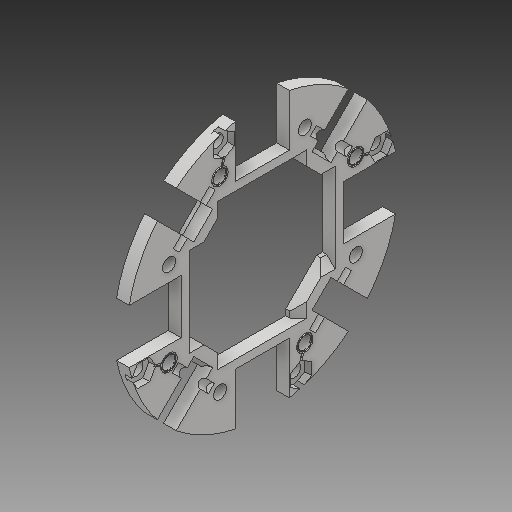
# Autodesk Inventor part: deska
Saved by Autodesk Inventor 2018 (Build 220112000, 112)
## iProperties
Created: 2018-03-10
Part Number: deska
Material: Všeobecné
Document SubType Name: Modeling
Designer: Kuba
Density: 1 g/cm^3
Appearance: Výchozí
Mass: 3.41348 g
Surface Area: 43.4622 cm^2
Volume: 3.41348 cm^3
Author: Kuba
Autodesk Inventor part; units mm, degrees
ref_plane "YZ Plane" through (0, 0, 0) normal (1, 0, 0) x (0, 1, 0)
sketch "Náčrt1" plane through (0, 0, 0) normal (1, 0, 0) x (0, 1, 0)
  line L0 (19.1636, 6.35) -> (31.3636, 6.35)
  line L1 (31.3636, -6.35) -> (19.1636, -6.35)
  line L2 (19.1636, -6.35) -> (19.1636, 6.35)
  line L3 (24.7449, 20.2901) -> (16.7231, 12.2683)
  line L4 (16.7231, 12.2683) -> (12.2683, 16.7231)
  line L5 (12.2683, 16.7231) -> (20.2901, 24.7449)
  line L6 (0, 0) -> (14.4957, 14.4957)
  line L7 (6.35, 19.1636) -> (-6.35, 19.1636)
  line L8 (6.35, 31.3636) -> (6.35, 19.1636)
  line L9 (-6.35, 19.1636) -> (-6.35, 31.3636)
  line L10 (-20.2901, 24.7449) -> (-12.2683, 16.7231)
  line L11 (-12.2683, 16.7231) -> (-16.7231, 12.2683)
  line L12 (-16.7231, 12.2683) -> (-24.7449, 20.2901)
  line L13 (-19.1636, 6.35) -> (-19.1636, -6.35)
  line L14 (-31.3636, 6.35) -> (-19.1636, 6.35)
  line L15 (-19.1636, -6.35) -> (-31.3636, -6.35)
  line L16 (-24.7449, -20.2901) -> (-16.7231, -12.2683)
  line L17 (-16.7231, -12.2683) -> (-12.2683, -16.7231)
  line L18 (-12.2683, -16.7231) -> (-20.2901, -24.7449)
  line L19 (-6.35, -19.1636) -> (6.35, -19.1636)
  line L20 (-6.35, -31.3636) -> (-6.35, -19.1636)
  line L21 (6.35, -19.1636) -> (6.35, -31.3636)
  line L22 (20.2901, -24.7449) -> (12.2683, -16.7231)
  line L23 (12.2683, -16.7231) -> (16.7231, -12.2683)
  line L24 (16.7231, -12.2683) -> (24.7449, -20.2901)
  arc A0 (24.7449, -20.2901) -> (31.3636, -6.35) centre (0, 0) ccw
  arc A1 (6.35, -31.3636) -> (20.2901, -24.7449) centre (0, 0) ccw
  arc A2 (-20.2901, -24.7449) -> (-6.35, -31.3636) centre (0, 0) ccw
  arc A3 (-31.3636, -6.35) -> (-24.7449, -20.2901) centre (0, 0) ccw
  arc A4 (-24.7449, 20.2901) -> (-31.3636, 6.35) centre (0, 0) ccw
  arc A5 (-6.35, 31.3636) -> (-20.2901, 24.7449) centre (0, 0) ccw
  arc A6 (31.3636, 6.35) -> (24.7449, 20.2901) centre (0, 0) ccw
  arc A7 (20.2901, 24.7449) -> (6.35, 31.3636) centre (0, 0) ccw
  line L25 (16.2792, 20.734) -> (20.734, 16.2792)
  line L26 (14.9711, 23.4564) -> (13.5569, 22.0421)
  line L27 (13.5569, 22.0421) -> (22.0421, 13.5569)
  line L28 (22.0421, 13.5569) -> (23.4564, 14.9711)
  line L29 (23.4564, 14.9711) -> (14.9711, 23.4564)
  line L30 (-13.5569, 22.0421) -> (-14.9711, 23.4564)
  line L31 (-22.0421, 13.5569) -> (-13.5569, 22.0421)
  line L32 (-14.9711, 23.4564) -> (-23.4564, 14.9711)
  line L33 (-23.4564, 14.9711) -> (-22.0421, 13.5569)
  line L34 (-22.0421, -13.5569) -> (-23.4564, -14.9711)
  line L35 (-13.5569, -22.0421) -> (-22.0421, -13.5569)
  line L36 (-23.4564, -14.9711) -> (-14.9711, -23.4564)
  line L37 (-14.9711, -23.4564) -> (-13.5569, -22.0421)
  line L38 (13.5569, -22.0421) -> (14.9711, -23.4564)
  line L39 (22.0421, -13.5569) -> (13.5569, -22.0421)
  line L40 (14.9711, -23.4564) -> (23.4564, -14.9711)
  line L41 (23.4564, -14.9711) -> (22.0421, -13.5569)
  line L42 (0, 0) -> (2.9116, 0)
  point P0 (-14.4957, 14.4957)
  point P1 (-14.4957, -14.4957)
  point P2 (14.4957, -14.4957)
  dimension "d1" = 6.35
  dimension "d2" = 6.35
  dimension "d4" = 6.3
  dimension "d5" = 3.15
  dimension "d6" = 20.5
  dimension "d7" = 45
  dimension "d10" = 360
  dimension "d12" = 2
  dimension "d13" = 12
  dimension "d14" = 1
  dimension "d15" = 2.85
  dimension "d18" = 360
  dimension "d105" = 32
  dimension "d106" = 45
  dimension "d107" = 12.2
  constraints: 86 end point, 16 point on circle, 8 centre point, 6 midpoint, 4 parallel, 3 perpendicular, 2 horizontal, 1 coincident, 94 other
  measures "d1" vertical distance of point (0, 0) L0.start
  measures "d2" distance from line of point (0, 0) L1
  measures "d4" distance between parallel lines of L3 L5
  measures "d5" distance between parallel lines of L6 L5
  measures "d6" distance from line of point (0, 0) L4
  measures "d7" angle of L2 L6
  measures "d12" distance of L26.start L26.end
  measures "d13" distance of L28.end L26.start
  measures "d14" distance between parallel lines of L25 L29
  measures "d15" distance between parallel lines of L5 L26
  measures "d105" radius of A5
  measures "d106" angle of L42 L6
  measures "d107" distance of L0.end L0.start
extrude "Vysunutí1" add sketch "Náčrt1" along normal mid plane 3 contours L2 L1 A0 L24 L40 L41 L39 L23 L22 L38 A1 L21 L19 L20 A2 L18 L36 L37 L35 L17 L16 L34 A3 L15 L13 L14 A4 L12 L32 L33 L31 L11 L10 L30 A5 L9 L7 L8 A7 L5 L29 L26 L27 L4 L3 L28 A6 L0 | L29 L28 L27 L3 | L5 L27 L26 L29 | L24 L39 L41 L40 | L40 L38 L39 L22 | L32 L30 L31 L10 | L12 L31 L33 L32 | L18 L35 L37 L36 | L36 L34 L35 L16
ref_plane "Pracovní rovina1" through (1.5, 0, 0) normal (1, 0, 0) x (0, 0, -1)
ref_plane "Pracovní rovina2" through (-1.5, 0, 0) normal (-1, 0, 0) x (0, 0, 1)
sketch "Náčrt6" plane through (-1.5, 0, 0) normal (1, 0, 0) x (0, 0, -1)
  circle A0 centre (10, 22) radius 1.3
  circle A1 centre (-10, 22) radius 1.3
  circle A2 centre (-22, 10) radius 1.3
  circle A3 centre (-22, -10) radius 1.3
  circle A4 centre (-10, -22) radius 1.3
  circle A5 centre (10, -22) radius 1.3
  circle A6 centre (22, -10) radius 1.3
  circle A7 centre (22, 10) radius 1.3
  point P0 (0, 0)
  dimension "d52" = 2.6
  dimension "d53" = 2.6
  dimension "d54" = 22
  dimension "d55" = 22
  dimension "d56" = 10
  dimension "d57" = 10
  dimension "d60" = 360
  constraints: 8 centre point, 17 other
  measures "d52" diameter of A0
  measures "d53" diameter of A1
  measures "d54" vertical distance of point (0, 0) A0.centre
  measures "d55" vertical distance of point (0, 0) A1.centre
  measures "d56" horizontal distance of point (0, 0) A0.centre
  measures "d57" horizontal distance of point (0, 0) A1.centre
sketch "Sketch7" plane through (-1.5, 16.7231, 12.2683) normal (0, -0.7071, 0.7071) x (1, 0, 0)
  circle A0 centre (2.9795, 2.3446) radius 1
  line L0 (0, 11.3446) -> (3, 11.3446) projected
  point P0 (1.5, -20.5)
  dimension "d64" = 2
  dimension "d65" = 9
  constraints: 1 centre point
  measures "d64" diameter of A0
  measures "d65" distance from line of L0 A0.centre
extrude "Extrusion6" cut sketch "Sketch7" against normal blind 3 and the other way blind 9
pattern_circular "Circular Pattern1" count 4 over 360 about axis through (0, 0, 0) along (1, 0, 0) of "Extrusion6"
hole "Hole3" at (-1.5, 10, 22) at (-1.5, 22, 10) at (-1.5, -10, 22) at (-1.5, -22, 10) at (-1.5, -22, -10) at (-1.5, 22, -10) at (-1.5, 10, -22) at (-1.5, -10, -22) direction (1, 0, 0) diameter 3.1 end through all countersink diameter 4.8 countersink angle 90
sketch "Sketch9" plane through (1.5, -20.2901, 24.7449) normal (0, -0.7071, -0.7071) x (-1, 0, 0)
  circle A0 centre (0.0205, 9) radius 3.15
  arc A1 (0, 8.0002) -> (0, 9.9998) centre (0.0205, 9) ccw projected
  point P0 (1.5, 31.8446)
  dimension "d102" = 6.3
  constraints: 1 centre point, 1 concentric
  measures "d102" diameter of A0
extrude "Extrusion7" cut sketch "Sketch9" along normal blind 6.3
pattern_circular "Circular Pattern2" count 4 over 360 about axis through (0, 0, 0) along (1, 0, 0) of "Extrusion7"
sketch "Sketch10" plane through (1.5, 0, 0) normal (1, 0, 0) x (0, 0, -1)
  line L0 (7.1094, 17.1636) -> (17.1636, 7.1094)
  line L1 (17.1636, 7.1094) -> (17.1636, -7.1094)
  line L2 (17.1636, -7.1094) -> (7.1094, -17.1636)
  line L3 (7.1094, -17.1636) -> (-7.1094, -17.1636)
  line L4 (-7.1094, -17.1636) -> (-17.1636, -7.1094)
  line L5 (-17.1636, -7.1094) -> (-17.1636, 7.1094)
  line L6 (-17.1636, 7.1094) -> (-7.1094, 17.1636)
  line L7 (-7.1094, 17.1636) -> (7.1094, 17.1636)
  line L8 (6.35, 19.1636) -> (-6.35, 19.1636) projected
  point P0 (0, 0)
  point P1 (0, 0)
  dimension "d111" = 2
  constraints: 16 end point, 1 coincident, 1 vertical, 17 other
  measures "d111" distance between parallel lines of L8 L7
extrude "Extrusion8" cut sketch "Sketch10" against normal blind 6.3
sketch "Sketch11" plane through (1.5, 0, 0) normal (1, 0, 0) x (0, 0, -1)
  line L0 (8.5, -17.1636) -> (-8.5, -17.1636)
  line L1 (-8.5, -17.1636) -> (-8.5, -7.1636)
  line L2 (-8.5, -7.1636) -> (8.5, -7.1636)
  line L3 (8.5, -7.1636) -> (8.5, -17.1636)
  line L4 (7.1094, -17.1636) -> (-7.1094, -17.1636) projected
  line L5 (0, 0) -> (0, -3.635)
  line L6 (0, 0) -> (-4.1702, 0)
  line L7 (17.1636, 8.5) -> (17.1636, -8.5)
  line L8 (17.1636, -8.5) -> (7.1636, -8.5)
  line L9 (7.1636, -8.5) -> (7.1636, 8.5)
  line L10 (7.1636, 8.5) -> (17.1636, 8.5)
  line L11 (-8.5, 17.1636) -> (8.5, 17.1636)
  line L12 (8.5, 17.1636) -> (8.5, 7.1636)
  line L13 (8.5, 7.1636) -> (-8.5, 7.1636)
  line L14 (-8.5, 7.1636) -> (-8.5, 17.1636)
  line L15 (-17.1636, -8.5) -> (-17.1636, 8.5)
  line L16 (-17.1636, 8.5) -> (-7.1636, 8.5)
  line L17 (-7.1636, 8.5) -> (-7.1636, -8.5)
  line L18 (-7.1636, -8.5) -> (-17.1636, -8.5)
  point P0 (3.635, 0)
  point P1 (0, 3.635)
  point P2 (-3.635, 0)
  dimension "d114" = 10
  dimension "d115" = 17
  dimension "d118" = 360
  constraints: 36 end point, 2 horizontal, 2 parallel, 1 collinear, 1 perpendicular, 1 vertical, 38 other
  measures "d114" distance between parallel lines of L2 L0
  measures "d115" distance of L0.start L0.end
extrude "Extrusion9" cut sketch "Sketch11" against normal through all contours L0 L1 L18 L17 L2 L9 L8 L3 | L8 L9 L2 L3 | L3 L2 L9 L13 L12 L10 L7 L8 | L18 L15 L16 L14 L13 L17 L2 L1 | L1 L2 L17 L18 | L13 L17 L16 L14 L11 L12 L10 L9 | L9 L10 L12 L13 | L13 L14 L16 L17
sketch "Sketch12" plane through (1.5, -17.1636, 8.5) normal (0, 1, 0) x (1, 0, 0)
  line L0 (0, 0) -> (0, -2)
  line L1 (0, -2) -> (-2, 0)
  line L2 (0, 0) -> (-3, 0) projected
  line L3 (-2, 0) -> (-3, 0)
  line L4 (-1.5, 8.5) -> (-3, 8.5)
  line L5 (-3, 0) -> (-3, 17) projected
  dimension "d123" = 2
  dimension "d129" = 45
  constraints: 8 end point, 3 point on line, 2 horizontal, 1 vertical
  measures "d123" distance of L0.start L0.end
  measures "d129" angle of L0 L1
extrude "Extrusion10" cut sketch "Sketch12" along normal up to surface (34.3273 mm away)
pattern_circular "Circular Pattern3" count 4 over 360 about axis through (0, 0, 0) along (1, 0, 0) of "Extrusion10"
sketch "Sketch14" plane through (1.5, 0, 0) normal (1, 0, 0) x (0, 0, -1)
  line L0 (25.1132, 9.1) -> (26.5566, 11.6)
  line L1 (26.5566, 11.6) -> (29.4434, 11.6)
  line L2 (29.4434, 11.6) -> (30.8868, 9.1)
  line L3 (30.8868, 9.1) -> (29.4434, 6.6)
  line L4 (29.4434, 6.6) -> (26.5566, 6.6)
  line L5 (26.5566, 6.6) -> (25.1132, 9.1)
  line L6 (19.1636, 6.35) -> (31.3636, 6.35) projected
  line L7 (-9.1, 25.1132) -> (-11.6, 26.5566)
  line L8 (-11.6, 26.5566) -> (-11.6, 29.4434)
  line L9 (-11.6, 29.4434) -> (-9.1, 30.8868)
  line L10 (-9.1, 30.8868) -> (-6.6, 29.4434)
  line L11 (-6.6, 29.4434) -> (-6.6, 26.5566)
  line L12 (-6.6, 26.5566) -> (-9.1, 25.1132)
  line L13 (-25.1132, -9.1) -> (-26.5566, -11.6)
  line L14 (-26.5566, -11.6) -> (-29.4434, -11.6)
  line L15 (-29.4434, -11.6) -> (-30.8868, -9.1)
  line L16 (-30.8868, -9.1) -> (-29.4434, -6.6)
  line L17 (-29.4434, -6.6) -> (-26.5566, -6.6)
  line L18 (-26.5566, -6.6) -> (-25.1132, -9.1)
  line L19 (9.1, -25.1132) -> (11.6, -26.5566)
  line L20 (11.6, -26.5566) -> (11.6, -29.4434)
  line L21 (11.6, -29.4434) -> (9.1, -30.8868)
  line L22 (9.1, -30.8868) -> (6.6, -29.4434)
  line L23 (6.6, -29.4434) -> (6.6, -26.5566)
  line L24 (6.6, -26.5566) -> (9.1, -25.1132)
  point P0 (0, 0)
  point P1 (28, 9.1)
  point P2 (-9.1, 28)
  point P3 (-28, -9.1)
  point P4 (9.1, -28)
  dimension "d140" = 9.1
  dimension "d141" = 28
  dimension "d142" = 5
  dimension "d145" = 360
  constraints: 48 end point, 1 parallel, 66 other
  measures "d140" vertical distance of point (28, 9.1) point (0, 0)
  measures "d141" horizontal distance of point (0, 0) point (28, 9.1)
  measures "d142" distance between parallel lines of L4 L1
extrude "Extrusion12" cut sketch "Sketch14" against normal blind 1.6
sketch "Sketch15" plane through (1.5, 0, 0) normal (1, 0, 0) x (0, 0, -1)
  circle A0 centre (22, 10) radius 1.65
  line L0 (25.2936, 8.7876) -> (23.5157, 9.3016)
  line L1 (23.5157, 9.3016) -> (23.6545, 9.7819)
  line L2 (23.6545, 9.7819) -> (25.4325, 9.268)
  line L3 (25.4325, 9.268) -> (25.2936, 8.7876)
  line L4 (22, 10) -> (23.3062, 9.6224)
  circle A1 centre (22, 10) radius 1.55 projected
  line L5 (26.5566, 6.6) -> (25.1132, 9.1) projected
  circle A2 centre (22, 10) radius 1.95
  point P0 (0, 0)
  dimension "d149" = 0.5
  dimension "d150" = 0.1
  dimension "d151" = 0.3
  constraints: 10 end point, 2 centre point, 2 parallel, 2 point on line, 1 coincident, 1 concentric, 1 perpendicular, 1 symmetric about line, 1 tangent
  measures "d149" distance of L0.end L1.end
  measures "d150" radial gap between concentric circles of A0 A1
  measures "d151" radial gap between concentric circles of A2 A0
extrude "Extrusion13" cut sketch "Sketch15" against normal blind 0.3 contours L1 L0 A2 L2 | L1 L2 A2 L0 | A2 L2 L3 L0
pattern_circular "Circular Pattern4" count 4 over 360 about axis through (0, 0, 0) along (1, 0, 0) of "Extrusion13"
sketch "Sketch16" plane through (-0.1, 0, 0) normal (1, 0, 0) x (0, 0, -1)
  circle A0 centre (28, 9.1) radius 2.8868
  circle A1 centre (-9.1, 28) radius 2.8868
  circle A2 centre (-28, -9.1) radius 2.8868
  circle A3 centre (9.1, -28) radius 2.8868
  point P0 (0, 0)
  point P1 (29.4434, 6.6)
  point P2 (29.4434, 11.6)
  point P3 (25.1132, 9.1)
  point P4 (-6.6, 29.4434)
  point P5 (-11.6, 29.4434)
  point P6 (-9.1, 25.1132)
  point P7 (-29.4434, -6.6)
  point P8 (-29.4434, -11.6)
  point P9 (-25.1132, -9.1)
  point P10 (6.6, -29.4434)
  point P11 (11.6, -29.4434)
  point P12 (9.1, -25.1132)
  dimension "d159" = 360
  constraints: 12 point on circle, 4 centre point, 21 other
hole "Hole4" at (-0.1, 28, 9.1) at (-0.1, -9.1, 28) at (-0.1, -28, -9.1) at (-0.1, 9.1, -28) direction (-1, 0, 0) diameter 3 end through all
equation "\"d2\" = d1"
equation "\"d5\" = 0.5 * d4"
equation "\"d14\" = 0.5 * d12"
equation "\"d15\" = -0.5 * d4 + 0.5 * d13"
equation "\"d55\" = d54"
equation "\"d57\" = d56"
equation "\"d36\" = 0.5 * d35"
equation "\"d35\" = 14"
